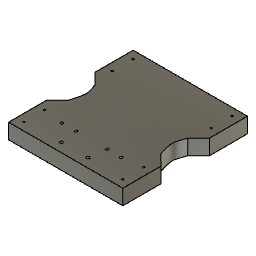
chassi 2.0 v1 (Autodesk Fusion 360 design; units mm, degrees)
Autodesk Fusion 360 part; units mm, degrees
sketch "Esboço1" plane through (0, 0, 0) normal (0, 0, 1) x (1, 0, 0)
  line L0 (-100, 200) -> (-100, 150)
  line L1 (-99.9888, 86.3572) -> (-99.9888, 36.3572)
  line L2 (-99.9888, 36.3572) -> (50.0112, 36.3572)
  line L3 (-100, 200) -> (50, 200)
  line L4 (50, 200) -> (50, 150)
  line L5 (50.0112, 36.3572) -> (50.0112, 86.3572)
  line L6 (-99.9888, 86.3572) -> (-85.8446, 100.4973)
  line L7 (50.0112, 86.3572) -> (35.8252, 100.4553)
  line L8 (50, 150) -> (35.8579, 135.8579)
  line L9 (-100, 150) -> (-85.8579, 135.8579)
  spline S0 degree 2 poles (-85.8446, 100.4973) (-80, 120) (-85.8579, 135.8579) knots 0 0 0 3.643978 3.643978 3.643978 weights 1 3 1
  spline S1 degree 2 poles (35.8252, 100.4553) (30, 120) (35.8579, 135.8579) knots 0 0 0 3.647748 3.647748 3.647748 weights 1 3 1
  dimension "d1" = 50
  dimension "d5" = 50
  dimension "d6" = 150
  dimension "d7" = 150
  dimension "d8" = 50
  dimension "d9" = 50
  dimension "d13" = 20
  dimension "d14" = 20
  dimension "d15" = 20
  dimension "d16" = 20
  constraint vertical L0
  constraint vertical L1
  constraint perpendicular L1 L2
  constraint perpendicular L0 L3
  constraint perpendicular L3 L4
  constraint perpendicular L2 L5
  measures "d1" distance of L0.start L0.end
  measures "d5" distance of L1.start L1.end
  measures "d6" distance of L1.end L2.end
  measures "d7" distance of L0.start L3.end
  measures "d8" distance of L3.end L4.end
  measures "d9" distance of L2.end L5.end
  measures "d13" distance of L1.start L6.end
  measures "d14" distance of L5.end L7.end
  measures "d15" distance of L4.end L8.end
  measures "d16" distance of L0.end L9.end
extrude "Extrusão1" add sketch "Esboço1" along normal blind 20
hole "Furo1" at (40, 190, 20) direction (0, 0, -1) diameter 2.5 depth 30 tip angle 118
hole "Furo2" at (40, 162.5, 20) direction (0, 0, -1) diameter 2.5 depth 30 tip angle 118
hole "Furo3" at (-90, 190, 20) direction (0, 0, -1) diameter 2.5 depth 30 tip angle 118
hole "Furo4" at (-90, 162.5, 20) direction (0, 0, -1) diameter 2.5 depth 30 tip angle 118
hole "Furo5" at (-89.9888, 73.8572, 20) direction (0, 0, -1) diameter 2.5 depth 30 tip angle 118
hole "Furo6" at (-89.9888, 46.3572, 20) direction (0, 0, -1) diameter 2.5 depth 30 tip angle 118
hole "Furo7" at (40.0112, 73.8572, 20) direction (0, 0, -1) diameter 2.5 depth 30 tip angle 118
hole "Furo8" at (40.0112, 46.3572, 20) direction (0, 0, -1) diameter 2.5 depth 30 tip angle 118
hole "Furo9" at (-42.4888, 48.3572, 20) direction (0, 0, -1) diameter 4 depth 30 tip angle 118
hole "Furo10" at (-7.4888, 48.3572, 20) direction (0, 0, -1) diameter 4 depth 30 tip angle 118
hole "Furo11" at (14.0112, 70.3572, 20) direction (0, 0, -1) diameter 3.5 depth 30 tip angle 118
hole "Furo12" at (-4.4888, 70.3572, 20) direction (0, 0, -1) diameter 3.5 depth 30 tip angle 118
hole "Furo13" at (-45.4888, 70.3572, 20) direction (0, 0, -1) diameter 3.5 depth 30 tip angle 118
hole "Furo14" at (-63.9888, 70.3572, 20) direction (0, 0, -1) diameter 3.5 depth 30 tip angle 118
